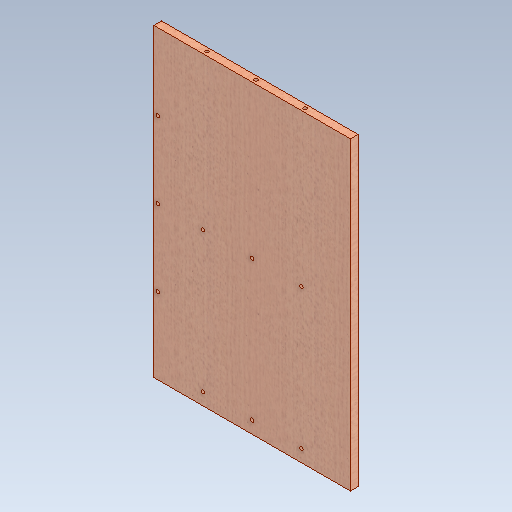
# Autodesk Inventor part: LateralMenor
Saved by Autodesk Inventor 2020.3 (Build 243373000, 373)
## iProperties
Created: 2020-10-27
Part Number: LateralMenor
Material: Madera (roble)
Document SubType Name: Modeling
Designer: codig
Density: 0.76 g/cm^3
Appearance: Roble blanco - Natural brillo medio
Author: codig
Autodesk Inventor part; units mm, degrees
ref_plane "YZ Plane" through (0, 0, 0) normal (1, 0, 0) x (0, 1, 0)
ref_plane "XZ Plane" through (0, 0, 0) normal (0, 1, 0) x (-1, 0, 0)
ref_plane "XY Plane" through (0, 0, 0) normal (0, 0, 1) x (1, 0, 0)
sketch "Boceto1" plane through (0, 0, 0) normal (0, 0, 1) x (1, 0, 0)
  line L0 (100, 100) -> (564, 100)
  line L1 (564, 100) -> (564, 820)
  line L2 (564, 820) -> (100, 820)
  line L3 (100, 820) -> (100, 100)
  point P0 (0, 0)
  constraints: 8 end point, 2 parallel, 1 horizontal, 1 perpendicular
extrude "Extrusión1" add sketch "Boceto1" along normal blind 18
sketch "Boceto2" plane through (100, 820, 0) normal (0, 1, 0) x (1, 0, 0)
  line L0 (464, 0) -> (464, -18) projected
  circle A0 centre (116, -9) radius 4
  circle A1 centre (232, -9) radius 4
  circle A2 centre (348, -9) radius 4
  point P0 (-100, 0)
  constraints: 3 centre point
hole "Agujero1" at (448, 820, 9) at (332, 820, 9) at (216, 820, 9) direction (0, -1, 0) diameter 8 depth 35
sketch "Boceto3" plane through (0, 0, 18) normal (0, 0, 1) x (1, 0, 0)
  circle A0 centre (109, 280) radius 4
  circle A1 centre (109, 460) radius 4
  circle A2 centre (109, 640) radius 4
  point P0 (0, 0)
  constraints: 3 centre point
hole "Agujero2" at (109, 280, 18) at (109, 460, 18) at (109, 640, 18) direction (0, 0, -1) diameter 8 depth 10
sketch "Boceto4" plane through (0, 0, 18) normal (0, 0, 1) x (1, 0, 0)
  circle A0 centre (216, 129) radius 4
  circle A1 centre (332, 129) radius 4
  circle A2 centre (448, 129) radius 4
  point P0 (0, 0)
  constraints: 3 centre point
hole "Agujero3" at (448, 129, 18) at (332, 129, 18) at (216, 129, 18) direction (0, 0, -1) diameter 8 depth 10
sketch "Boceto5" plane through (0, 0, 18) normal (0, 0, 1) x (1, 0, 0)
  line L0 (100, 820) -> (100, 100) projected
  line L1 (564, 100) -> (564, 820) projected
  circle A0 centre (332, 129) radius 4 projected
  circle A1 centre (332, 460) radius 4
  circle A2 centre (448, 129) radius 4 projected
  circle A3 centre (448, 460) radius 4
  circle A4 centre (216, 129) radius 4 projected
  circle A5 centre (216, 460) radius 4
  point P0 (0, 0)
  constraints: 3 centre point
hole "Agujero4" at (448, 460, 18) at (332, 460, 18) at (216, 460, 18) direction (0, 0, -1) diameter 8 depth 10
sketch "Boceto6" plane through (100, 100, 0) normal (0, -1, 0) x (1, 0, 0)
  circle A0 centre (116, 9) radius 4
  circle A1 centre (232, 9) radius 4
  circle A2 centre (348, 9) radius 4
  point P0 (-100, 0)
  constraints: 3 centre point
hole "Agujero5" at (448, 100, 9) at (332, 100, 9) at (216, 100, 9) direction (0, 1, 0) diameter 8 depth 23
